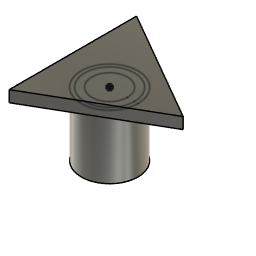
with_switch (Autodesk Fusion 360 archive; units mm, degrees)
design "table_design_1"
Autodesk Fusion 360 part; units mm, degrees
sketch "Sketch2" plane through (0, 0, 0) normal (0, 0, 1) x (1, 0, 0)
  line L0 (519.6152, 0) -> (-259.8076, 450)
  line L1 (-259.8076, 450) -> (-259.8076, -450)
  line L2 (-259.8076, -450) -> (519.6152, 0)
  dimension "d4" = 900
  measures "d4" distance of L0.start L0.end
extrude "Extrude2" add sketch "Sketch2" along normal blind 80
sketch "Sketch3" plane through (0, 0, 0) normal (0, 0, 1) x (1, 0, 0)
  circle A0 centre (0, 0) radius 125
  circle A1 centre (0, 0) radius 200
  circle A2 centre (0, 0) radius 175
  dimension "d7" = 250
  dimension "d8" = 400
  dimension "d9" = 350
  constraint coincident A0.centre A1.centre
  measures "d7" diameter of A0
  measures "d8" diameter of A1
  measures "d9" diameter of A2
extrude "Extrude3" add sketch "Sketch3" against normal blind 200 contours A0
extrude "Extrude4" add sketch "Sketch3" against normal blind 500 contours A1
extrude "Extrude5" cut 1 faces at (62.6805, -21.2553, -200) along direction (0, 0, 1) blind 200
extrude "Extrude6" add sketch "Sketch3" against normal blind 400 contours A0
extrude "Extrude7" cut 1 faces at (190.2705, -18.6303, -500) along direction (0, 0, 1) blind 100
extrude "Extrude8" add 1 faces at (190.2705, -18.6303, -400) along direction (0, 0, -1) blind 50
